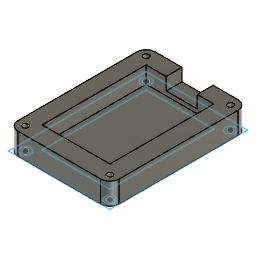
Jackson's ATK (Autodesk Fusion 360 design; units mm, degrees)
part number: 2025-12-03-21-45-55-105
part number: 2025-12-03-21-49-20-157
Autodesk Fusion 360 part; units mm, degrees
sketch "Sketch1" plane through (0, 0, 0) normal (0, 0, 1) x (1, 0, 0) in component "Jackson's Editing ATK"
  line L0 (-33.4351, 34.2031) -> (6.9349, 34.2031)
  line L1 (6.9349, 34.2031) -> (6.9349, 96.1631)
  line L2 (6.9349, 96.1631) -> (-33.4351, 96.1631)
  line L3 (-33.4351, 96.1631) -> (-33.4351, 34.2031)
  line L4 (-42.9351, 105.6631) -> (17.4349, 105.6631)
  line L5 (17.4349, 105.6631) -> (17.4349, 23.7031)
  line L6 (17.4349, 23.7031) -> (-42.9351, 23.7031)
  line L7 (-42.9351, 23.7031) -> (-42.9351, 105.6631)
  circle A0 centre (-37.9351, 28.7031) radius 1.7
  circle A1 centre (-37.9351, 28.7031) radius 3
  circle A2 centre (12.4349, 28.7031) radius 1.7
  circle A3 centre (12.4349, 28.7031) radius 1.7
  circle A4 centre (12.4349, 28.7031) radius 3
  circle A5 centre (12.4349, 100.6631) radius 1.7
  circle A6 centre (12.4349, 100.6631) radius 3
  circle A7 centre (-37.9351, 100.6631) radius 1.7
  circle A8 centre (-37.9351, 100.6631) radius 3
  dimension "d1" = 61.96
  dimension "d2" = 40.37
  dimension "d3" = 60.37
  dimension "d4" = 81.96
  dimension "d5" = 9.5
  dimension "d6" = 9.5
  dimension "d7" = 3.4
  dimension "d8" = 5
  dimension "d9" = 5
  dimension "d17" = 6
  dimension "d20" = 3.4
  dimension "d21" = 5
  dimension "d22" = 5
  dimension "d23" = 3.4
  dimension "d24" = 6
  dimension "d25" = 3.4
  dimension "d26" = 5
  dimension "d27" = 5
  dimension "d28" = 6
  dimension "d29" = 3.4
  dimension "d30" = 5
  dimension "d31" = 5
  dimension "d32" = 6
  constraint horizontal L0
  constraint vertical L1
  constraint horizontal L2
  constraint vertical L3
  constraint horizontal L4
  constraint vertical L5
  constraint horizontal L6
  constraint vertical L7
  constraint coincident A0.centre A1.centre
  constraint coincident A2.centre A3.centre
  constraint coincident A5.centre A6.centre
  constraint coincident A7.centre A8.centre
  measures "d1" distance of L0.start L2.end
  measures "d2" distance of L0.start L0.end
  measures "d3" distance of L5.end L6.end
  measures "d4" distance of L4.end L5.end
  measures "d5" distance of L2 L4
  measures "d6" distance of L3 L7
  measures "d7" diameter of A0
  measures "d8" distance of L6 A0.centre
  measures "d9" distance of L7 A0.centre
  measures "d17" diameter of A1
  measures "d20" diameter of A2
  measures "d21" distance of L6 A2.centre
  measures "d22" distance of L5 A2.centre
  measures "d23" diameter of A3
  measures "d24" diameter of A4
  measures "d25" diameter of A5
  measures "d26" distance of L4 A5.centre
  measures "d27" distance of L5 A5.centre
  measures "d28" diameter of A6
  measures "d29" diameter of A7
  measures "d30" distance of L4 A7.centre
  measures "d31" distance of L7 A7.centre
  measures "d32" diameter of A8
extrude "Extrude1" add sketch "Sketch1" along normal blind 9.9 from surface at 3.1 contours A1 | A4 | A6 | A8 makes body 1 at (-34.9388, 28.5536, 9.7) makes body 2 at (-35.3752, 102.2274, 9.7) makes body 3 at (15.4312, 28.5536, 9.7) makes body 4 at (15.254, 99.6371, 9.7) in component "Jackson's Editing ATK"
extrude "Extrude2" add sketch "Sketch1" along normal blind 13 contours L4 L5 L6 L7 bodies 1 2 3 4 in component "Jackson's Editing ATK"
extrude "Extrude3" add sketch "Sketch1" along normal blind 3 contours L0 L1 L2 L3 bodies 1 in component "Jackson's Editing ATK"
sketch "Sketch2" plane through (0, 0, 13) normal (0, 0, 1) x (-1, 0, 0) in component "Jackson's Editing ATK"
  circle A0 centre (37.9351, -28.7031) radius 1.7
  circle A1 centre (-12.4349, -100.6631) radius 1.7
  line L0 (33.4351, -34.2031) -> (33.4351, -96.1631)
  line L1 (33.4351, -96.1631) -> (-6.9349, -96.1631)
  line L2 (-6.9349, -96.1631) -> (-6.9349, -34.2031)
  line L3 (-6.9349, -34.2031) -> (33.4351, -34.2031)
  line L4 (42.9351, -23.7031) -> (-17.4349, -23.7031)
  line L5 (-17.4349, -23.7031) -> (-17.4349, -105.6631)
  line L6 (-17.4349, -105.6631) -> (42.9351, -105.6631)
  line L7 (42.9351, -105.6631) -> (42.9351, -23.7031)
  circle A2 centre (37.9351, -100.6631) radius 1.7
  circle A3 centre (-12.4349, -28.7031) radius 1.7
  line L8 (21.4871, -96.1631) -> (2.9871, -96.1631)
  line L9 (2.9871, -96.1631) -> (2.9871, -105.6631)
  line L10 (2.9871, -105.6631) -> (21.4871, -105.6631)
  line L11 (21.4871, -105.6631) -> (21.4871, -96.1631)
  dimension "d40" = 21.448
  dimension "d41" = 18.5
  constraint horizontal L8
  constraint vertical L9
  constraint horizontal L10
  constraint vertical L11
  constraint coincident L6 L9.end
  constraint coincident L1 L8.start
  measures "d40" distance of L7 L11
  measures "d41" distance of L8.start L8.end
extrude "Extrude4" cut sketch "Sketch2" against normal blind 7.5 contours L1 L6 L8 L9 L10 L11 bodies 1 in component "Jackson's Editing ATK"
fillet "Fillet1" radius 5.5 1 edges at (-42.9351, 23.7031, 6.5) on bodies 1 in component "Jackson's Editing ATK"
fillet "Fillet2" radius 5.5 1 edges at (17.4349, 23.7031, 6.5) on bodies 1 in component "Jackson's Editing ATK"
fillet "Fillet3" radius 5.5 1 edges at (17.4349, 105.6631, 6.5) on bodies 1 in component "Jackson's Editing ATK"
fillet "Fillet4" radius 5.5 1 edges at (-42.9351, 105.6631, 6.5) on bodies 1 in component "Jackson's Editing ATK"
component "Jackson's Editing ATK" placed x (1, 0, 0) y (0, 1, 0) z (0, 0, 1) at (0, 0, 0)
